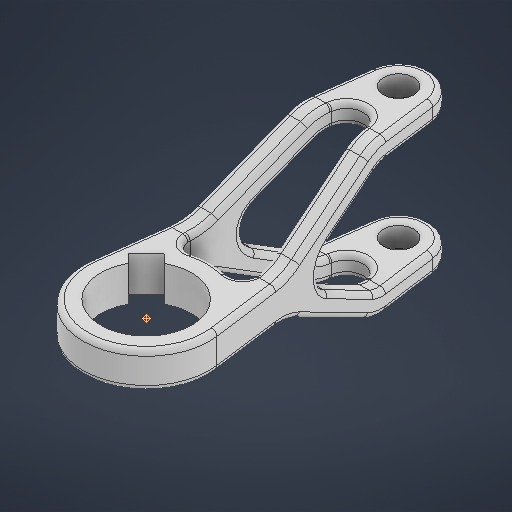
# Autodesk Inventor part: b2
Saved by Autodesk Inventor 2025.4 (Build 294407000, 407)
## iProperties
Created: 2026-05-15
Part Number: b2
Material: Generic
Document SubType Name: Modeling
Designer: VuQuan
Density: 1 g/cm^3
Appearance: Default
Author: VuQuan
Autodesk Inventor part; units mm, degrees
ref_plane "YZ Plane" through (0, 0, 0) normal (1, 0, 0) x (0, 1, 0)
ref_plane "XZ Plane" through (0, 0, 0) normal (0, 1, 0) x (-1, 0, 0)
ref_plane "XY Plane" through (0, 0, 0) normal (0, 0, 1) x (1, 0, 0)
sketch "Sketch1" plane through (0, 0, 0) normal (0, 1, 0) x (-1, 0, 0)
  line L0 (0, 0) -> (0, -100) construction
  line L1 (24.7878, -3.25) -> (11.8982, -101.56)
  arc A0 (-11.8982, -101.56) -> (11.8982, -101.56) centre (0, -100) ccw
  line L2 (-11.8982, -101.56) -> (-24.7878, -3.25)
  arc A1 (24.7878, -3.25) -> (-24.7878, -3.25) centre (0, 0) ccw
  circle A2 centre (0, -100) radius 6
  arc A3 (15.7626, -8.6915) -> (8.6915, -15.7626) centre (0, 0) ccw
  line L3 (15.7626, -8.6915) -> (19.0919, -12.0208)
  line L4 (19.0919, -12.0208) -> (12.0208, -19.0919)
  line L5 (12.0208, -19.0919) -> (8.6915, -15.7626)
  line L6 (15.5563, -15.5563) -> (0, 0) construction
  line L7 (0, 0) -> (18, 0) construction
  line L8 (13.1399, -30.5507) -> (6.6329, -80.18)
  arc A4 (-6.6329, -80.18) -> (6.6329, -80.18) centre (0, -79.3103) ccw
  line L9 (-6.6329, -80.18) -> (-13.1399, -30.5507)
  arc A5 (-6.8626, -25.078) -> (-13.1399, -30.5507) centre (-8.1824, -29.9007) ccw
  arc A6 (-6.8626, -25.078) -> (6.8626, -25.078) centre (0, 0) ccw
  arc A7 (13.1399, -30.5507) -> (6.8626, -25.078) centre (8.1824, -29.9007) ccw
  point P0 (-12.7279, 12.7279)
  point P1 (-12.7279, 12.7279)
  point P2 (0, -86)
  point P3 (0, -94)
  dimension "d3" = 12
  dimension "d0" = 100
  dimension "d1" = 25
  dimension "d2" = 12
  dimension "d4" = 36
  dimension "d5" = 45
  dimension "d6" = 10
  dimension "d7" = 40
  dimension "d8" = 8
  dimension "d9" = 8
  dimension "d10" = 5
  dimension "d11" = 8
  constraints: 20 end point, 18 point on circle, 10 tangent, 7 centre point, 5 coincident, 4 perpendicular, 3 point on line, 2 parallel, 1 equal radius, 1 midpoint, 1 vertical, 1 vertical alignment, 2 other
  measures "d0" distance of L0.start L0.end
  measures "d1" radius of A1
  measures "d2" radius of A0
  measures "d4" diameter of A3
  measures "d5" angle of L6 L7
  measures "d6" distance of L3.end L4.end
  measures "d7" distance from line of point (-12.728, 12.728) L4
  measures "d8" radial gap between concentric circles of A3 A6
  measures "d9" distance between parallel lines of L1 L8
  measures "d10" radius of A7
  measures "d11" distance of point (0, -94) point (0, -86)
extrude "Extrusion1" add sketch "Sketch1" along normal mid plane 60
sketch "Sketch2" plane through (0, 0, 0) normal (1, 0, 0) x (0, 1, 0)
  line L0 (0, 25) -> (-7, 25)
  line L1 (-7, 25) -> (-7, -29.6599)
  arc A0 (-9.6619, -39.6293) -> (-7, -29.6599) centre (-27, -29.6599) ccw
  line L2 (-9.6619, -39.6293) -> (-27.6043, -70.8336)
  arc A1 (-27.6043, -70.8336) -> (-30, -79.8061) centre (-12, -79.8061) ccw
  line L3 (-30, -79.8061) -> (-30, -112)
  line L4 (-30, -112) -> (-22, -112)
  line L5 (-22, -112) -> (-22, -79.8061)
  arc A2 (-20.6691, -74.8214) -> (-22, -79.8061) centre (-12, -79.8061) ccw
  line L6 (-20.6691, -74.8214) -> (-8.6691, -53.9518)
  arc A3 (0, -48.9365) -> (-8.6691, -53.9518) centre (0, -58.9365) ccw
  line L7 (0, 25) -> (0, -48.9365) construction
  line L8 (30, -3.25) -> (30, 25) projected
  line L9 (30, -3.25) -> (30, -101.56) projected
  line L10 (30, -112) -> (30, -101.56) projected
  line L11 (0, 25) -> (7, 25)
  line L12 (7, 25) -> (7, -29.6599)
  arc A4 (7, -29.6599) -> (9.6619, -39.6293) centre (27, -29.6599) ccw
  line L13 (9.6619, -39.6293) -> (27.6043, -70.8336)
  arc A5 (30, -79.8061) -> (27.6043, -70.8336) centre (12, -79.8061) ccw
  line L14 (30, -79.8061) -> (30, -112)
  line L15 (22, -112) -> (22, -79.8061)
  line L16 (20.6691, -74.8214) -> (8.6691, -53.9518)
  arc A6 (30, -79.8061) -> (27.6043, -70.8336) centre (12, -79.8061) ccw
  line L17 (30, -112) -> (22, -112)
  arc A7 (22, -79.8061) -> (20.6691, -74.8214) centre (12, -79.8061) ccw
  arc A8 (8.6691, -53.9518) -> (0, -48.9365) centre (0, -58.9365) ccw
  point P0 (0, 0)
  point P1 (-30, -75)
  point P2 (-7, -35)
  point P3 (7, -35)
  point P4 (30, -79.8061)
  dimension "d14" = 10
  dimension "d15" = 20
  dimension "d16" = 14
  dimension "d17" = 10
  dimension "d18" = 8
  dimension "d19" = 60
  dimension "d21" = 35
  dimension "d22" = 75
  constraints: 30 end point, 18 point on circle, 14 symmetric about line, 10 point on line, 9 centre point, 7 tangent, 3 perpendicular, 2 coincident, 2 parallel, 1 horizontal, 1 vertical, 5 other
  measures "d14" radius of A2
  measures "d15" radius of A0
  measures "d16" diameter of L1 L7
  measures "d17" radius of A3
  measures "d18" distance between parallel lines of L3 L5
  measures "d19" diameter of L3 L7
  measures "d21" vertical distance of point (-7, -35) point (0, 0)
  measures "d22" vertical distance of point (-30, -75) point (0, 0)
extrude "Extrusion2" cut sketch "Sketch2" along normal through all both and the other way through all keep common part
fillet "Fillet1" radius 2 84 edges at (20.6487, 7.6769, -34.8193) (17.9724, 18.6331, -55.2315) (15.3592, 29.3908, -75.1627) (13.3243, 30, -90.683) (0, 30, -112) (-13.3243, 30, -90.683) (-15.3592, 29.3908, -75.1627) (-17.9724, 18.6331, -55.2315) (-20.6487, 7.6769, -34.8193) (-23.0565, 7, -16.455) (0, 7, 25) (23.0565, 7, -16.455) (0, -7, 25) (-23.0565, -7, -16.455) (-20.6487, -7.6769, -34.8193) (-17.9724, -18.6331, -55.2315) (-15.3592, -29.3908, -75.1627) (-13.3243, -30, -90.683) (0, -30, -112) (13.3243, -30, -90.683) (15.3592, -29.3908, -75.1627) (17.9724, -18.6331, -55.2315) (20.6487, -7.6769, -34.8193) (23.0565, -7, -16.455) (0, -22, -112) (-13.3243, -22, -90.683) (-15.0886, -21.6615, -77.2264) (-16.7721, -14.6691, -64.3866) (-18.6215, -5.0076, -50.2807) (-16.7721, 14.6691, -64.3866) (-15.0886, 21.6615, -77.2264) (-13.3243, 22, -90.683) (0, 22, -112) (13.3243, 22, -90.683) (15.0886, 21.6615, -77.2264) (16.7721, 14.6691, -64.3866) (18.6215, -5.0076, -50.2807) (16.7721, -14.6691, -64.3866) (15.0886, -21.6615, -77.2264) (13.3243, -22, -90.683) (-11.119, 7, -25.8539) (-13.1781, 7.005, -30.1071) (-12.524, 7.7966, -35.2484) (-9.904, 18.6331, -55.2315) (-7.2907, 29.3908, -75.1627) (-6.6574, 30, -79.993) (0, 30, -86) (6.6574, 30, -79.993) (7.2907, 29.3908, -75.1627) (9.904, 18.6331, -55.2315) (12.524, 7.7966, -35.2484) (13.1781, 7.005, -30.1071) (11.119, 7, -25.8539) (0, 7, -26) (-12.524, -7.7966, -35.2484) (-13.1781, -7.005, -30.1071) (-11.119, -7, -25.8539) (0, -7, -26) (11.119, -7, -25.8539) (13.1781, -7.005, -30.1071) (12.524, -7.7966, -35.2484) (9.904, -18.6331, -55.2315) (7.2907, -29.3908, -75.1627) (6.6574, -30, -79.993) (0, -30, -86) (-6.6574, -30, -79.993) (-7.2907, -29.3908, -75.1627) (-9.904, -18.6331, -55.2315) (6.6574, -22, -79.993) (7.0201, -21.6615, -77.2264) (8.7036, -14.6691, -64.3866) (10.5531, -5.0076, -50.2807) (8.7036, 14.6691, -64.3866) (7.0201, 21.6615, -77.2264) (6.6574, 22, -79.993) (0, 22, -86) (-6.6574, 22, -79.993) (-7.0201, 21.6615, -77.2264) (-8.7036, 14.6691, -64.3866) (-10.5531, -5.0076, -50.2807) (-8.7036, -14.6691, -64.3866) (-7.0201, -21.6615, -77.2264) (-6.6574, -22, -79.993) (0, -22, -86)
body "Solid1"
